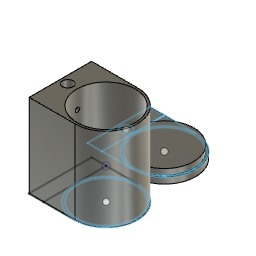
Motor Holder small v1 v1 (Autodesk Fusion 360 design; units mm, degrees)
Autodesk Fusion 360 part; units mm, degrees
sketch "Sketch2" plane through (0, 0, 0) normal (0, 0, 1) x (1, 0, 0)
  line L0 (0, 0) -> (0, -30)
  circle A0 centre (15, -15) radius 15
  line L1 (0, -30) -> (15, -30)
  line L2 (0, 0) -> (15, 0)
  line L3 (0, -30) -> (-7, -30)
  line L4 (-7, -30) -> (-7, 0)
  line L5 (-7, 0) -> (0, 0)
  circle A1 centre (15, -15) radius 0.5
  dimension "d1" = 30
  dimension "d2" = 30
  dimension "d3" = 7
  dimension "d4" = 1
  constraint coincident L0.start L2.start
  constraint vertical L0
  constraint coincident A0 L1.end
  constraint tangent A0 L1
  constraint perpendicular L0 L1
  constraint coincident A0 L2.end
  constraint tangent A0 L2
  constraint perpendicular L0 L2
  constraint perpendicular L0 L3
  constraint perpendicular L3 L4
  constraint perpendicular L4 L5
  constraint concentric A0 A1
  measures "d1" distance of L0.start L0.end
  measures "d2" diameter of A0
  measures "d3" distance of L0.end L3.end
  measures "d4" diameter of A1
extrude "Extrude1" add sketch "Sketch2" along normal blind 40 makes body 1
sketch "Sketch3" plane through (0, 0, 0) normal (0, 0, 1) x (1, 0, 0)
  circle A0 centre (15, -15) radius 14
  dimension "d7" = 28
  measures "d7" diameter of A0
hole "Hole1" at (15, -15, 40) direction (0, 0, -1) diameter 28 depth 38 tip angle 180 bodies 1
form "Form1" [no effect]
fillet "Fillet1" radius 0.5 1 edges at (1.9474, -9.9374, 2) on bodies 1
hole "Hole2" at (-7, -14.7821, 31.1998) direction (1, 0, 0) diameter 2 depth 9 tip angle 180 bodies 1
hole "Hole3" at (-3.3751, -15.0621, 40) direction (0, 0, -1) diameter 5 depth 5 tip angle 180 bodies 1
sketch "Sketch4" plane through (0, 0, 0) normal (0, 0, 1) x (1, 0, 0)
  line L0 (-7, 5) -> (-7, 35)
  circle A0 centre (8, 20) radius 15
  line L1 (-7, 35) -> (8, 35)
  line L2 (-7, 5) -> (8, 5)
  line L3 (-7, 5) -> (-14, 5)
  line L4 (-14, 5) -> (-14, 35)
  line L5 (-14, 35) -> (-7, 35)
  circle A1 centre (8, 20) radius 14.05
  circle A2 centre (-10.3753, 19.9378) radius 2.55
  dimension "d19" = 30
  dimension "d20" = 30
  dimension "d21" = 7
  dimension "d22" = 28.1
  dimension "d30" = 5.1
  constraint vertical L0
  constraint coincident A0 L1.end
  constraint tangent A0 L1
  constraint coincident A0 L2.end
  constraint tangent A0 L2
  constraint perpendicular L0 L3
  constraint perpendicular L3 L4
  constraint concentric A0 A1
  measures "d19" distance of L0.start L0.end
  measures "d20" diameter of A0
  measures "d21" distance of L0.start L3.end
  measures "d22" diameter of A1
  measures "d30" diameter of A2
sketch "Sketch6" plane through (0, 0, 0) normal (0, 0, 1) x (1, 0, 0)
extrude "Extrude5" add sketch "Sketch4" against normal blind 3 separate body contours L0 L3 L4 L5 | L0 A0 L2 | L0 A0 L1 | A0 | A1 | A2 makes body 2
extrude "Extrude6" add sketch "Sketch4" along normal blind 5 contours A2 bodies 2
extrude "Extrude7" add sketch "Sketch4" along normal blind 2.8 contours A1 bodies 2
extrude "Extrude2" [rolled back] along distance 3 taper angle 0
extrude "Extrude3" [rolled back] along distance -2.8 taper angle 0
sketch "Sketch5" plane through (0, 0, 0) normal (0, 0, 1) x (1, 0, 0)
  circle A0 centre (-10.5005, 19.9379) radius 2.5
  dimension "d27" = 5
  measures "d27" diameter of A0
extrude "Extrude4" [rolled back] along distance -5 taper angle 0
sketch "Sketch1" plane through (0, 0, 0) normal (0, 0, 1) x (1, 0, 0)
  line L0 (0, 0) -> (0, -50)
  constraint coincident L0.start origin
  constraint vertical L0
